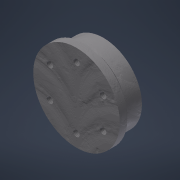
# Autodesk Inventor part: BridaTornillo2
Saved by Autodesk Inventor 2022 (Build 260153000, 153)
## iProperties
Created: 2021-09-22
Part Number: BridaTornillo2
Material: Steel, Mild, Welded
Document SubType Name: Modeling
Designer: Andres
Density: 7.85 g/cm^3
Appearance: Weld - Steel Mild
Mass: 118.114 g
Surface Area: 58.6184 cm^2
Volume: 15.0463 cm^3
Author: Andres
Autodesk Inventor part; units mm, degrees
ref_plane "YZ Plane" through (0, 0, 0) normal (1, 0, 0) x (0, 1, 0)
ref_plane "XZ Plane" through (0, 0, 0) normal (0, 1, 0) x (-1, 0, 0)
sketch "Sketch1" plane through (0, 0, 0) normal (0, 0, 1) x (1, 0, 0)
  point P0 (0, 0)
sketch "Sketch2" plane through (0, 0, 0) normal (0, 0, 1) x (1, 0, 0)
  circle A0 centre (0, 0) radius 20
  line L0 (-5.1962, -3) -> (5.1962, -3) projected
  arc A1 (5.1962, -3) -> (-5.1962, -3) centre (0, 0) ccw projected
  point P0 (0, 0)
  dimension "d26" = 40
  constraints: 1 centre point
  measures "d26" diameter of A0
extrude "Extrusion1" add sketch "Sketch2" against normal blind 10 contours A0 | A1 L0
sketch "Sketch3" plane through (0, 0, 0) normal (0, 0, 1) x (1, 0, 0)
  circle A0 centre (0, 0) radius 22.5
  dimension "d4" = 45
  constraints: 1 centre point, 1 coincident
  measures "d4" diameter of A0
extrude "Extrusion2" add sketch "Sketch3" along normal blind 4
ref_plane "Work Plane1" through (0.1016, -6, 79.4067) normal (0, -1, 0) x (1, 0, 0)
sketch "Sketch4" plane through (0.1016, -6, 79.4067) normal (0, -1, 0) x (1, 0, 0)
  arc A0 (1.3984, -81.4067) -> (-1.6016, -81.4067) centre (-0.1016, -81.4067) ccw projected
  line L0 (-1.6016, -81.4067) -> (-1.6016, -87.4067) projected
  line L1 (1.3984, -87.4067) -> (1.3984, -81.4067) projected
  arc A1 (-1.6016, -87.4067) -> (1.3984, -87.4067) centre (-0.1016, -87.4067) ccw projected
  line L2 (-1.6016, -87.4067) -> (-1.6016, -88.4067)
  line L3 (-1.6016, -88.4067) -> (1.3984, -88.4067)
  line L4 (1.3984, -88.4067) -> (1.3984, -87.4067)
  line L5 (-20.1016, -89.4067) -> (19.8984, -89.4067) projected
  point P0 (-0.1016, -79.4067)
  point P1 (7.8984, -88.7552)
  point P2 (-8.1016, -88.7552)
  point P3 (1.5, -80.6705)
  point P4 (-1.5, -80.6705)
  point P5 (-1.6016, -86.4323)
  point P6 (1.0165, -88.4067)
  point P7 (-1.2196, -88.4067)
  constraints: 6 end point, 1 collinear, 1 parallel, 1 perpendicular, 1 point on circle
extrude "Extrusion3" [suppressed]
sketch "Sketch5" plane through (0, 0, 0) normal (0, 0, -1) x (-1, 0, 0)
  circle A0 centre (0, 0) radius 22.5 projected
  circle A1 centre (0, 0) radius 20 projected
chamfer "Chamfer2" distance 2 angle 45 1 edges at (-20, 0, 0)
sketch "Sketch6" plane through (0, 0, 4) normal (0, 0, 1) x (1, 0, 0)
  circle A0 centre (0, 0) radius 16 construction
  point P0 (0, 16)
  dimension "d15" = 32
  constraints: 2 vertical alignment, 1 coincident, 2 other
hole "Hole1" at (0, 16, 4) direction (0, 0, -1) diameter 3.242 depth 11 tip angle 118 thread size "M4x0.7" class "6H" standard "ISO Metric profile"
pattern_circular "Circular Pattern1" count 6 over 360 about axis through (0, 0, 0) along (0, 0, 1) of "Hole1"
sketch "Sketch7" plane through (0, 0, -10) normal (0, 0, -1) x (-1, 0, 0)
  line L0 (7.4162, -3) -> (-7.4162, -3) projected
  circle A0 centre (0, 0) radius 8 projected
  point P0 (0, 0)
extrude "Extrusion4" cut sketch "Sketch7" against normal blind 10 contours L0 A0 picked at (2.2034, 0.3877)
chamfer "Chamfer3" distance 2 angle 45 1 edges at (0, 8, 0)
body "Solid1"
